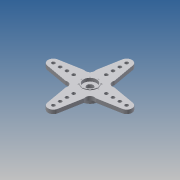
# Autodesk Inventor part: 4-PRONG SERVO ARM ONYX
Saved by Autodesk Inventor 2022.1 (Build 261234000, 234)
## iProperties
Created: 2021-08-13
Part Number: 4-PRONG SERVO ARM ONYX
Material: Nylon 6/6
Document SubType Name: Modeling
Designer: dotwibo2
Mass: 0.28903 g
Surface Area: 4.66998 cm^2
Volume: 0.255779 cm^3
Density: 1.13 g/cm^3
Appearance: White
Author: dotwibo2
Autodesk Inventor part; units mm, degrees
ref_plane "YZ Plane" through (0, 0, 0) normal (1, 0, 0) x (0, 1, 0)
ref_plane "XZ Plane" through (0, 0, 0) normal (0, 1, 0) x (-1, 0, 0)
ref_plane "XY Plane" through (0, 0, 0) normal (0, 0, 1) x (1, 0, 0)
sketch "Sketch1" plane through (0, 0, 0) normal (0, 0, 1) x (1, 0, 0)
  line L0 (0, -4.462) -> (0, 3.322) projected
  line L1 (3.05, 2.21) -> (3.05, 0.71)
  line L2 (3.05, 0.71) -> (1.5, 0.71)
  line L3 (1.5, 0.71) -> (1.5, -0.35)
  line L4 (1.5, -0.35) -> (2.925, -0.35)
  line L5 (2.925, -0.35) -> (2.925, -3.35)
  line L6 (2.925, -3.35) -> (4, -3.35)
  line L7 (4, -3.35) -> (4, 0)
  line L8 (4, 0) -> (6, 0)
  line L9 (6, 0) -> (6, 1.8)
  line L10 (6, 1.8) -> (3.5, 1.8)
  line L11 (3.5, 1.8) -> (3.5, 2.21)
  line L12 (3.5, 2.21) -> (3.05, 2.21)
  line L13 (-1.2, 0) -> (7.2, 0) construction
  point P0 (0, 0)
  dimension "d1" = 5.85
  dimension "d2" = 3
  dimension "d3" = 5.56
  dimension "d4" = 1.5
  dimension "d5" = 6.1
  dimension "d6" = 7
  dimension "d7" = 8
  dimension "d8" = 1.8
  dimension "d9" = 3.35
  dimension "d10" = 12
  dimension "d20" = 3
  constraints: 24 end point, 6 horizontal, 6 vertical, 1 collinear
  measures "d1" diameter of L5 L0
  measures "d2" diameter of L3 L0
  measures "d3" distance between parallel lines of L6 L12
  measures "d4" distance between parallel lines of L12 L2
  measures "d5" diameter of L1 L0
  measures "d6" diameter of L11 L0
  measures "d7" diameter of L7 L0
  measures "d8" distance between parallel lines of L8 L10
  measures "d9" distance between parallel lines of L8 L6
  measures "d10" diameter of L9 L0
  measures "d20" distance between parallel lines of L6 L4
revolve "Revolution1" add sketch "Sketch1" angle 360 about axis through (0, -10, 0) along (0, 1, 0)
fillet "Fillet1" radius 1 1 edges at (-4, 0, 0)
sketch "Sketch2" plane through (0, 0, 0) normal (0, 0, 1) x (1, 0, 0)
  line L0 (-3.05, 2.21) -> (3.05, 2.21) construction
  line L1 (-3.5, 2.21) -> (3.5, 2.21) construction
  line L2 (-3.5, 1.8) -> (3.5, 1.8) construction
  line L3 (-6, 1.8) -> (6, 1.8) construction
  line L4 (3.4965, 2.21) -> (4.2066, 1.8)
  line L5 (4.2066, 1.8) -> (3.4965, 1.8)
  line L6 (3.4965, 1.8) -> (3.4965, 2.21)
  point P0 (0, 0)
  dimension "d13" = 0.0035
  dimension "d14" = 60
  constraints: 6 end point, 3 point on line, 1 vertical
  measures "d13" distance from line of L1.end L6
  measures "d14" angle of L6 L4
extrude "Extrusion1" add sketch "Sketch2" along normal mid plane 0.3
pattern_circular "Circular Pattern1" count 8 over 360 about axis through (0, -10, 0) along (0, 1, 0) of "Extrusion1"
sketch "Sketch3" plane through (0, 0, 0) normal (0, 1, 0) x (-1, 0, 0)
  line L0 (-4.3493, 7.0069) -> (-2.4607, 17.5268)
  arc A0 (2.4607, 17.5268) -> (-2.4607, 17.5268) centre (0, 17.085) ccw
  line L1 (2.4607, 17.5268) -> (4.3493, 7.0069)
  line L2 (8.4, 0) -> (-8.4, 0) construction
  line L3 (0, -10.4993) -> (0, 20.9956) construction
  line L4 (-4.25, 7.56) -> (4.25, 7.56) construction
  arc A1 (3.9598, 3.9598) -> (-3.9598, 3.9598) centre (0, 0) ccw
  arc A2 (4.3493, 7.0069) -> (4.7977, 4.7977) centre (6.2407, 6.2407) ccw
  arc A3 (-4.7977, 4.7977) -> (-4.3493, 7.0069) centre (-6.2407, 6.2407) ccw
  line L5 (0, 0) -> (6.2407, 6.2407) construction
  line L6 (3.6956, 5.8998) -> (6.4334, 3.1621) construction
  line L7 (-4.2, 7.1075) -> (-4.2, 5.2789) construction
  line L8 (4.2, 7.1509) -> (4.2, 5.2556) construction
  line L9 (4.7977, 4.7977) -> (3.9598, 3.9598)
  line L10 (-4.7977, 4.7977) -> (-3.9598, 3.9598)
  point P0 (0, 7.56)
  point P1 (0, 13.91)
  point P2 (0, 10.735)
  dimension "d21" = 17.085
  dimension "d22" = 5
  dimension "d23" = 9.525
  dimension "d25" = 8.5
  dimension "d26" = 5.6
  dimension "d29" = 3.175
  dimension "d30" = 3.175
  dimension "d38" = 45
  dimension "d40" = 6.785
  dimension "d41" = 8.4
  constraints: 18 end point, 8 point on circle, 5 tangent, 4 centre point, 4 point on line, 2 coincident, 2 collinear, 2 vertical, 1 horizontal, 1 midpoint, 1 perpendicular, 3 other
  measures "d21" distance from line of L2 A0.centre
  measures "d22" diameter of A0
  measures "d23" distance of point (0, 7.56) A0.centre
  measures "d25" distance of L4.start L4.end
  measures "d26" radius of A1
  measures "d29" distance of point (0, 17.085) point (0, 13.91)
  measures "d30" distance of point (0, 10.735) point (0, 13.91)
  measures "d38" angle of L3 L5
  measures "d40" distance from line of point (0, 0) L6
  measures "d41" distance between parallel lines of L8 L7
extrude "Extrusion2" add sketch "Sketch3" along normal up to surface (1.8 mm away)
hole "Hole1" at (0, 0, 7.56) at (0, 0, 17.085) at (0, 0, 13.91) at (0, 0, 10.735) direction (0, 1, 0) diameter 1.6 end through all
pattern_circular "Circular Pattern2" count 4 over 360 about axis through (0, -10, 0) along (0, 1, 0) of "Extrusion2", "Hole1"
equation "\"d29\" = 0.333333 * d23"
equation "\"d30\" = d29"
body "Solid1"
